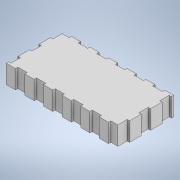
# Autodesk Inventor part: FrontPanel
Saved by Autodesk Inventor 2020.4 (Build 244396010, 396A)
## iProperties
Created: 2021-10-02
Part Number: FrontPanel
Material: Generic
Document SubType Name: Modeling
Designer: YUSTE
Density: 1 g/cm^3
Appearance: Default
Author: YUSTE
Autodesk Inventor part; units mm, degrees
ref_plane "YZ Plane" through (0, 0, 0) normal (1, 0, 0) x (0, 1, 0)
ref_plane "XZ Plane" through (0, 0, 0) normal (0, 1, 0) x (-1, 0, 0)
ref_plane "XY Plane" through (0, 0, 0) normal (0, 0, 1) x (1, 0, 0)
sketch "Sketch1" plane through (0, 0, 0) normal (0, 1, 0) x (-1, 0, 0)
  line L0 (0, 0) -> (0, 76.2)
  line L1 (0, 76.2) -> (152.4, 76.2)
  line L2 (152.4, 76.2) -> (152.4, 0)
  line L3 (152.4, 0) -> (0, 0)
  line L4 (139.7, 76.2) -> (127, 76.2)
  line L5 (127, 76.2) -> (127, 73.025)
  line L6 (127, 73.025) -> (139.7, 73.025)
  line L7 (139.7, 73.025) -> (139.7, 76.2)
  line L8 (114.3, 76.2) -> (101.6, 76.2)
  line L9 (101.6, 76.2) -> (101.6, 73.025)
  line L10 (101.6, 73.025) -> (114.3, 73.025)
  line L11 (114.3, 73.025) -> (114.3, 76.2)
  line L12 (88.9, 76.2) -> (76.2, 76.2)
  line L13 (76.2, 76.2) -> (76.2, 73.025)
  line L14 (76.2, 73.025) -> (88.9, 73.025)
  line L15 (88.9, 73.025) -> (88.9, 76.2)
  line L16 (63.5, 76.2) -> (50.8, 76.2)
  line L17 (50.8, 76.2) -> (50.8, 73.025)
  line L18 (50.8, 73.025) -> (63.5, 73.025)
  line L19 (63.5, 73.025) -> (63.5, 76.2)
  line L20 (38.1, 76.2) -> (25.4, 76.2)
  line L21 (25.4, 76.2) -> (25.4, 73.025)
  line L22 (25.4, 73.025) -> (38.1, 73.025)
  line L23 (38.1, 73.025) -> (38.1, 76.2)
  line L24 (12.7, 76.2) -> (0, 76.2)
  line L25 (0, 76.2) -> (0, 73.025)
  line L26 (0, 73.025) -> (12.7, 73.025)
  line L27 (12.7, 73.025) -> (12.7, 76.2)
  line L28 (152.4, 0) -> (139.7, 0)
  line L29 (139.7, 0) -> (139.7, 3.175)
  line L30 (139.7, 3.175) -> (152.4, 3.175)
  line L31 (152.4, 3.175) -> (152.4, 0)
  line L32 (127, 0) -> (114.3, 0)
  line L33 (114.3, 0) -> (114.3, 3.175)
  line L34 (114.3, 3.175) -> (127, 3.175)
  line L35 (127, 3.175) -> (127, 0)
  line L36 (101.6, 0) -> (88.9, 0)
  line L37 (88.9, 0) -> (88.9, 3.175)
  line L38 (88.9, 3.175) -> (101.6, 3.175)
  line L39 (101.6, 3.175) -> (101.6, 0)
  line L40 (76.2, 0) -> (63.5, 0)
  line L41 (63.5, 0) -> (63.5, 3.175)
  line L42 (63.5, 3.175) -> (76.2, 3.175)
  line L43 (76.2, 3.175) -> (76.2, 0)
  line L44 (50.8, 0) -> (38.1, 0)
  line L45 (38.1, 0) -> (38.1, 3.175)
  line L46 (38.1, 3.175) -> (50.8, 3.175)
  line L47 (50.8, 3.175) -> (50.8, 0)
  line L48 (25.4, 0) -> (12.7, 0)
  line L49 (12.7, 0) -> (12.7, 3.175)
  line L50 (12.7, 3.175) -> (25.4, 3.175)
  line L51 (25.4, 3.175) -> (25.4, 0)
  line L52 (152.4, 73.025) -> (149.225, 73.025)
  line L53 (149.225, 73.025) -> (149.225, 60.325)
  line L54 (149.225, 60.325) -> (152.4, 60.325)
  line L55 (152.4, 60.325) -> (152.4, 73.025)
  line L56 (152.4, 44.45) -> (149.225, 44.45)
  line L57 (149.225, 44.45) -> (149.225, 31.75)
  line L58 (149.225, 31.75) -> (152.4, 31.75)
  line L59 (152.4, 31.75) -> (152.4, 44.45)
  line L60 (152.4, 15.875) -> (149.225, 15.875)
  line L61 (149.225, 15.875) -> (149.225, 3.175)
  line L62 (149.225, 3.175) -> (152.4, 3.175)
  line L63 (152.4, 3.175) -> (152.4, 15.875)
  line L64 (0, 73.025) -> (0, 60.325)
  line L65 (0, 60.325) -> (3.175, 60.325)
  line L66 (3.175, 60.325) -> (3.175, 73.025)
  line L67 (3.175, 73.025) -> (0, 73.025)
  line L68 (0, 3.175) -> (0, 15.875)
  line L69 (0, 15.875) -> (3.175, 15.875)
  line L70 (3.175, 15.875) -> (3.175, 3.175)
  line L71 (3.175, 3.175) -> (0, 3.175)
  line L72 (0, 31.75) -> (0, 44.45)
  line L73 (0, 44.45) -> (3.175, 44.45)
  line L74 (3.175, 44.45) -> (3.175, 31.75)
  line L75 (3.175, 31.75) -> (0, 31.75)
  point P0 (149.225, 3.175)
  dimension "d176" = 76.2
  dimension "d177" = 152.4
  dimension "d178" = 12.7
  dimension "d179" = 3.175
  dimension "d180" = 12.7
  dimension "d181" = 12.7
  dimension "d182" = 3.175
  dimension "d183" = 12.7
  dimension "d184" = 3.175
  dimension "d185" = 12.7
  dimension "d186" = 3.175
  dimension "d187" = 12.7
  dimension "d188" = 3.175
  dimension "d189" = 12.7
  dimension "d190" = 12.7
  dimension "d191" = 12.7
  dimension "d192" = 12.7
  dimension "d193" = 12.7
  dimension "d194" = 3.175
  dimension "d195" = 12.7
  dimension "d196" = 12.7
  dimension "d197" = 3.175
  dimension "d198" = 12.7
  dimension "d199" = 3.175
  dimension "d200" = 12.7
  dimension "d201" = 3.175
  dimension "d202" = 12.7
  dimension "d203" = 3.175
  dimension "d204" = 12.7
  dimension "d205" = 12.7
  dimension "d206" = 12.7
  dimension "d207" = 12.7
  dimension "d208" = 3.175
  dimension "d209" = 12.7
  dimension "d210" = 3.175
  dimension "d211" = 12.7
  dimension "d212" = 12.7
  dimension "d213" = 3.175
  dimension "d214" = 12.7
  dimension "d215" = 3.175
  dimension "d216" = 3.175
  dimension "d217" = 12.7
  dimension "d218" = 15.875
  dimension "d219" = 3.175
  dimension "d220" = 12.7
  dimension "d222" = 3.175
  dimension "d223" = 12.7
  dimension "d224" = 3.175
  dimension "d225" = 12.7
  dimension "d226" = 3.175
  dimension "d227" = 3.175
  dimension "d228" = 12.7
  dimension "d229" = 3.175
  dimension "d230" = 15.875
  constraints: 148 end point, 37 parallel, 21 perpendicular, 8 point on line, 2 vertical, 29 other
  measures "d176" distance of L0.start L0.end
  measures "d177" distance of L0.end L2.start
  measures "d178" distance of L4.start L4.end
  measures "d179" distance of L5.end L4.end
  measures "d180" distance between parallel lines of L2 L7
  measures "d181" distance of L8.start L8.end
  measures "d182" distance of L9.end L8.end
  measures "d183" distance of L12.start L12.end
  measures "d184" distance of L13.end L12.end
  measures "d185" distance of L16.start L16.end
  measures "d186" distance of L17.end L16.end
  measures "d187" distance of L20.start L20.end
  measures "d188" distance of L21.end L20.end
  measures "d189" distance between parallel lines of L5 L11
  measures "d190" distance between parallel lines of L15 L9
  measures "d191" distance between parallel lines of L19 L13
  measures "d192" distance between parallel lines of L23 L17
  measures "d193" distance of L24.start L24.end
  measures "d194" distance of L25.end L24.end
  measures "d195" distance between parallel lines of L27 L21
  measures "d196" distance of L2.end L28.end
  measures "d197" distance of L28.end L29.end
  measures "d198" distance of L32.start L32.end
  measures "d199" distance of L32.end L33.end
  measures "d200" distance of L36.start L36.end
  measures "d201" distance of L36.end L37.end
  measures "d202" distance of L40.start L40.end
  measures "d203" distance of L40.end L41.end
  measures "d204" distance between parallel lines of L35 L29
  measures "d205" distance between parallel lines of L39 L33
  measures "d206" distance between parallel lines of L43 L37
  measures "d207" distance of L44.start L44.end
  measures "d208" distance of L44.end L45.end
  measures "d209" distance of L48.start L48.end
  measures "d210" distance of L48.end L49.end
  measures "d211" distance between parallel lines of L47 L41
  measures "d212" distance between parallel lines of L51 L45
  measures "d213" distance of L52.start L52.end
  measures "d214" distance of L53.end L52.end
  measures "d215" length of L52
  measures "d216" distance of L56.start L56.end
  measures "d217" distance of L57.end L56.end
  measures "d218" distance between parallel lines of L54 L56
  measures "d219" distance of L60.start L60.end
  measures "d220" distance of L61.end L60.end
  measures "d222" length of L62
  measures "d223" distance of L25.end L64.end
  measures "d224" distance of L65.end L64.end
  measures "d225" distance of L68.start L68.end
  measures "d226" distance of L68.end L69.end
  measures "d227" length of L71
  measures "d228" distance of L72.start L72.end
  measures "d229" distance of L72.end L73.end
  measures "d230" distance between parallel lines of L69 L75
extrude "Extrusion5" add sketch "Sketch1" along normal blind 25.4 contours L0 L71 L70 L69 L75 L74 L73 L65 L66 L26 L27 L1 L21 L22 L23 L17 L18 L19 L13 L14 L15 L9 L10 L11 L5 L6 L7 L2 L52 L53 L54 L56 L57 L58 L60 L61 L30 L29 L3 L35 L34 L33 L39 L38 L37 L43 L42 L41 L47 L46 L45 L51 L50 L49
body "Solid5"
